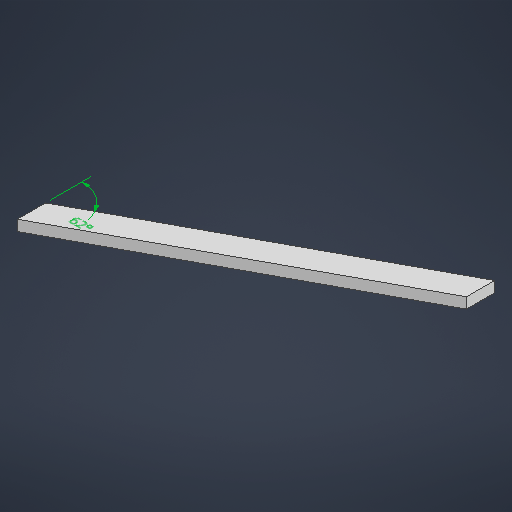
# Autodesk Inventor part: S_2x4x50.56
Saved by Autodesk Inventor 2027.1 (Build 311270010, 270A)
## iProperties
Created: 2026-09-01
Part Number: S_2x4x50.56
Material: Generic
Document SubType Name: Modeling
Designer: jorda
Density: 1 g/cm^3
Appearance: Default
Author: jorda
Autodesk Inventor part; units mm, degrees
ref_plane "YZ Plane" through (0, 0, 0) normal (1, 0, 0) x (0, 1, 0)
ref_plane "XZ Plane" through (0, 0, 0) normal (0, 1, 0) x (-1, 0, 0)
ref_plane "XY Plane" through (0, 0, 0) normal (0, 0, 1) x (1, 0, 0)
sketch "Sketch1" plane through (0, 0, 0) normal (0, 1, 0) x (-1, 0, 0)
  line L0 (187.2803, -609.6) -> (1041.4, -148.9512)
  line L1 (187.2803, -609.6) -> (0, -710.6051)
  line L2 (0, -710.6051) -> (0, -609.6)
  line L3 (1041.4, -47.9461) -> (0, -609.6)
  line L4 (1041.4, -47.9461) -> (1041.4, -148.9512)
  line L5 (1041.4, -148.9512) -> (184.524, -611.0865)
  point P0 (0, 0)
  constraints: 12 end point, 1 point on line, 1 vertical
extrude "Extrusion1" add sketch "Sketch1" along normal blind 38.1
body "Solid1"
